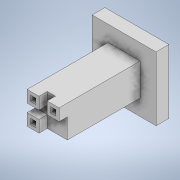
# Autodesk Inventor part: final_beam_cube
Saved by Autodesk Inventor 2021 (Build 250183000, 183)
## iProperties
Created: 2021-06-14
Part Number: final_beam_cube
Material: Generic
Document SubType Name: Modeling
Designer: user
Density: 1 g/cm^3
Appearance: Default
Author: user
Autodesk Inventor part; units mm, degrees
ref_plane "YZ Plane" through (0, 0, 0) normal (1, 0, 0) x (0, 1, 0)
ref_plane "XZ Plane" through (0, 0, 0) normal (0, 1, 0) x (-1, 0, 0)
ref_plane "XY Plane" through (0, 0, 0) normal (0, 0, 1) x (1, 0, 0)
sketch "Sketch1" plane through (0, 0, 0) normal (0, 0, 1) x (1, 0, 0)
  line L0 (-47.9977, 34.7826) -> (52.0023, 34.7826)
  line L1 (52.0023, 34.7826) -> (52.0023, -65.2174)
  line L2 (52.0023, -65.2174) -> (-47.9977, -65.2174)
  line L3 (-47.9977, -65.2174) -> (-47.9977, 34.7826)
  point P0 (0, 0)
  dimension "d0" = 100
  dimension "d1" = 100
  dimension "d2" = 100
  constraints: 8 end point, 2 parallel, 1 horizontal, 1 perpendicular
  measures "d0" distance of L0.start L0.end
  measures "d1" distance of L2.end L0.start
  measures "d2" distance of L1.end L2.end
extrude "Extrusion1" add sketch "Sketch1" along normal blind 20
sketch "Sketch2" plane through (0, 0, 20) normal (0, 0, 1) x (1, 0, 0)
  line L0 (-22.9977, 9.7826) -> (27.0023, 9.7826)
  line L1 (27.0023, 9.7826) -> (27.0023, -40.2174)
  line L2 (27.0023, -40.2174) -> (-22.9977, -40.2174)
  line L3 (-22.9977, -40.2174) -> (-22.9977, 9.7826)
  line L4 (52.0023, 34.7826) -> (-47.9977, 34.7826) projected
  line L5 (-47.9977, 34.7826) -> (-47.9977, -65.2174) projected
  line L6 (-47.9977, -65.2174) -> (52.0023, -65.2174) projected
  line L7 (52.0023, -65.2174) -> (52.0023, 34.7826) projected
  point P0 (0, 0)
  dimension "d5" = 25
  dimension "d6" = 25
  dimension "d7" = 25
  dimension "d8" = 25
  constraints: 8 end point, 2 parallel, 1 horizontal, 1 perpendicular
  measures "d5" distance between parallel lines of L4 L0
  measures "d6" distance between parallel lines of L5 L3
  measures "d7" distance between parallel lines of L6 L2
  measures "d8" distance between parallel lines of L7 L1
extrude "Extrusion2" add sketch "Sketch2" along normal blind 100 contours L0 L1 L2 L3
shell "Shell1" thickness 10 removed faces 1 at (-6.331, -6.8841, 120)
sketch "Sketch3" plane through (0, 0, 120) normal (0, 0, 1) x (1, 0, 0)
  line L0 (-22.9977, 9.7826) -> (-22.9977, -40.2174) projected
  line L1 (27.0023, -40.2174) -> (27.0023, 9.7826) projected
  line L2 (-22.9977, 9.7826) -> (27.0023, 9.7826)
  line L3 (27.0023, 9.7826) -> (27.0023, -40.2174)
  line L4 (27.0023, -40.2174) -> (-22.9977, -40.2174)
  line L5 (-22.9977, -40.2174) -> (-22.9977, 9.7826)
  point P0 (0, 0)
  constraints: 8 end point, 2 parallel, 1 horizontal, 1 perpendicular
extrude "Extrusion3" add sketch "Sketch3" along normal blind 13.65
sketch "Sketch4" plane through (0, 0, 133.65) normal (0, 0, 1) x (1, 0, 0)
  line L0 (-22.9977, 9.7826) -> (-4.3577, 9.7826)
  line L1 (-4.3577, 9.7826) -> (-4.3577, -8.8574)
  line L2 (-4.3577, -8.8574) -> (-22.9977, -8.8574)
  line L3 (-22.9977, -8.8574) -> (-22.9977, 9.7826)
  line L4 (27.0023, 9.7826) -> (8.3623, 9.7826)
  line L5 (8.3623, 9.7826) -> (8.3623, -8.8574)
  line L6 (8.3623, -8.8574) -> (27.0023, -8.8574)
  line L7 (27.0023, -8.8574) -> (27.0023, 9.7826)
  line L8 (27.0023, -40.2174) -> (-22.9977, -40.2174) projected
  line L9 (-22.9977, -40.2174) -> (-4.3577, -40.2174)
  line L10 (-4.3577, -40.2174) -> (-4.3577, -21.5774)
  line L11 (-4.3577, -21.5774) -> (-22.9977, -21.5774)
  line L12 (-22.9977, -21.5774) -> (-22.9977, -40.2174)
  point P0 (0, 0)
  dimension "d14" = 18.64
  dimension "d15" = 18.64
  dimension "d16" = 18.64
  dimension "d17" = 18.64
  dimension "d18" = 18.64
  constraints: 24 end point, 6 parallel, 3 horizontal, 3 perpendicular, 2 point on line
  measures "d14" distance of L1.end L2.end
  measures "d15" distance of L0.end L1.end
  measures "d16" distance of L5.end L6.end
  measures "d17" distance of L10.end L11.end
  measures "d18" distance of L9.end L10.end
extrude "Extrusion4" add sketch "Sketch4" along normal blind 12.8
sketch "Sketch5" plane through (0, 0, 146.45) normal (0, 0, 1) x (1, 0, 0)
  line L0 (13.3623, 4.7826) -> (22.0023, 4.7826)
  line L1 (22.0023, 4.7826) -> (22.0023, -3.8574)
  line L2 (22.0023, -3.8574) -> (13.3623, -3.8574)
  line L3 (13.3623, -3.8574) -> (13.3623, 4.7826)
  line L4 (-17.9977, 4.7826) -> (-9.3577, 4.7826)
  line L5 (-9.3577, 4.7826) -> (-9.3577, -3.8574)
  line L6 (-9.3577, -3.8574) -> (-17.9977, -3.8574)
  line L7 (-17.9977, -3.8574) -> (-17.9977, 4.7826)
  line L8 (-17.9977, -26.5774) -> (-9.3577, -26.5774)
  line L9 (-9.3577, -26.5774) -> (-9.3577, -35.2174)
  line L10 (-9.3577, -35.2174) -> (-17.9977, -35.2174)
  line L11 (-17.9977, -35.2174) -> (-17.9977, -26.5774)
  line L12 (-4.3577, 9.7826) -> (-22.9977, 9.7826) projected
  line L13 (-22.9977, 9.7826) -> (-22.9977, -8.8574) projected
  line L14 (-22.9977, -8.8574) -> (-4.3577, -8.8574) projected
  line L15 (-4.3577, -8.8574) -> (-4.3577, 9.7826) projected
  line L16 (27.0023, 9.7826) -> (8.3623, 9.7826) projected
  line L17 (27.0023, -8.8574) -> (27.0023, 9.7826) projected
  line L18 (8.3623, 9.7826) -> (8.3623, -8.8574) projected
  line L19 (-4.3577, -21.5774) -> (-22.9977, -21.5774) projected
  line L20 (-22.9977, -40.2174) -> (-4.3577, -40.2174) projected
  point P0 (0, 0)
  dimension "d21" = 5
  dimension "d22" = 5
  dimension "d23" = 5
  dimension "d24" = 5
  dimension "d25" = 5
  dimension "d26" = 5
  dimension "d27" = 5
  dimension "d28" = 5
  dimension "d29" = 5
  constraints: 24 end point, 6 parallel, 4 point on line, 3 horizontal, 3 perpendicular
  measures "d21" distance between parallel lines of L12 L4
  measures "d22" distance between parallel lines of L13 L7
  measures "d23" distance between parallel lines of L14 L6
  measures "d24" distance between parallel lines of L15 L5
  measures "d25" distance between parallel lines of L16 L0
  measures "d26" distance between parallel lines of L17 L1
  measures "d27" distance between parallel lines of L18 L3
  measures "d28" distance between parallel lines of L19 L8
  measures "d29" distance between parallel lines of L20 L10
extrude "Extrusion5" cut sketch "Sketch5" against normal blind 15 contours L0 L1 L2 L3 | L4 L5 L6 L7 | L8 L9 L10 L11
equation "\"d1\" = d0"
equation "\"d6\" = d5"
equation "\"d7\" = d5"
equation "\"d8\" = d5"
equation "\"d15\" = d14"
equation "\"d16\" = d14"
equation "\"d18\" = d14"
equation "\"d22\" = d21"
equation "\"d23\" = d21"
equation "\"d24\" = d21"
equation "\"d26\" = d21"
equation "\"d27\" = d21"
equation "\"d28\" = d21"
equation "\"d29\" = d21"
body "Solid1"
